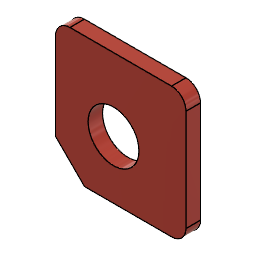
base plate 2 (Autodesk Fusion 360 design; units mm, degrees)
part number: 2025-11-19-20-55-22-502
Autodesk Fusion 360 part; units mm, degrees
sketch "Sketch1" plane through (0, 0, 0) normal (0, 0, 1) x (1, 0, 0)
  line L0 (0, 0) -> (80, 0)
  line L1 (90, 10) -> (90, 80)
  line L2 (80, 90) -> (10, 90)
  line L3 (0, 80) -> (0, 0)
  line L4 (0, 20) -> (20, 0)
  circle A0 centre (40, 40) radius 17.5
  arc A1 (10, 90) -> (0, 80) centre (10, 80) ccw
  arc A2 (90, 80) -> (80, 90) centre (80, 80) ccw
  arc A3 (80, 0) -> (90, 10) centre (80, 10) ccw
  point P0 (90, 0)
  point P1 (0, 90)
  dimension "d1" = 90
  dimension "d2" = 90
  dimension "d3" = 20
  dimension "d4" = 20
  dimension "d5" = 35
  dimension "d6" = 40
  dimension "d7" = 40
  dimension "d8" = 10
  dimension "d9" = 10
  dimension "d10" = 10
  constraint horizontal L0
  constraint vertical L1
  constraint horizontal L2
  constraint vertical L3
  constraint coincident L0.start L3.end
  constraint coincident L3 L4.start
  constraint coincident L0 L4.end
  constraint coincident P1 L2
  constraint coincident P1 L3
  constraint tangent L2 A1
  constraint tangent L3 A1
  constraint tangent L1 A2
  constraint tangent L2 A2
  constraint coincident P0 L0
  constraint coincident P0 L1
  constraint tangent L0 A3
  constraint tangent L1 A3
  measures "d1" distance of L0.start P0
  measures "d2" distance of L0.start P1
  measures "d3" distance of L0.start L4.start
  measures "d4" distance of L0.start L4.end
  measures "d5" diameter of A0
  measures "d6" distance of L3 A0.centre
  measures "d7" distance of L0 A0.centre
  measures "d8" radius of A1
  measures "d9" radius of A2
  measures "d10" radius of A3
extrude "Extrude1" add sketch "Sketch1" along normal blind 10 contours L0 L1 L2 L3 L4 A1 A2 A3
